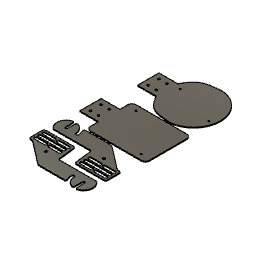
DécoupeCNC (Autodesk Fusion 360 design; units mm, degrees)
Autodesk Fusion 360 part; units mm, degrees
sketch "Esquisse2" plane through (0, 0, 0) normal (0, 0, 1) x (1, 0, 0) in component "Support Joystick v4"
  line L0 (0, 0) -> (-70, 0)
  circle A0 centre (100, 0) radius 82.5
  line L1 (250, 0) -> (-130, 0)
  spline S0 degree 5 poles (0, 20) (0, 22.4882) (0.1779, 27.4114) (0.975, 34.6277) (3.4457, 44.3914) (10.1068, 57.8847) (21.3924, 73.1358) (35.9935, 85.4932) (52.8737, 92.6951) (72.095, 96.3693) (93.5882, 98.471) (117.0022, 100.5708) (140.5192, 100.2508) (161.4884, 92.9068) (178.6566, 78.1832) (191.1793, 56.7401) (197.2314, 35.6259) (199.4965, 18.2943) (200, 6.1899) (200, 0) knots 0 0 0 0 0 0 0.066667 0.133333 0.2 0.266667 0.333333 0.4 0.466667 0.533333 0.6 0.666667 0.733333 0.8 0.866667 0.933333 1 1 1 1 1 1
  line L2 (0, 0) -> (0, 40)
  line L3 (96.4605, 99.786) -> (143.5395, 100.214)
  line L4 (4.3857, 52.2523) -> (35.6143, 87.7477)
  spline S1 degree 5 poles (0, -20) (0, -22.4882) (0.1779, -27.4114) (0.975, -34.6277) (3.4457, -44.3914) (10.1068, -57.8847) (21.3924, -73.1358) (35.9935, -85.4932) (52.8737, -92.6951) (72.095, -96.3693) (93.5882, -98.471) (117.0022, -100.5708) (140.5192, -100.2508) (161.4884, -92.9068) (178.6566, -78.1832) (191.1793, -56.7401) (197.2314, -35.6259) (199.4965, -18.2943) (200, -6.1899) (200, 0) knots 0 0 0 0 0 0 0.066667 0.133333 0.2 0.266667 0.333333 0.4 0.466667 0.533333 0.6 0.666667 0.733333 0.8 0.866667 0.933333 1 1 1 1 1 1
  line L5 (200, 30) -> (200, -30)
  line L6 (0, 0) -> (0, -40)
  line L7 (4.3857, -52.2523) -> (35.6143, -87.7477)
  line L8 (96.4605, -99.786) -> (143.5395, -100.214)
  line L9 (200, -30) -> (200, 30)
  circle A1 centre (22.2756, 27.6617) radius 3.1
  circle A2 centre (179.3345, -22.6338) radius 3.1
  ellipse E0 centre (100, 0) end of major axis (100, 100) minor radius 100
  line L10 (100, -100) -> (100, 100)
  line L11 (200, 0) -> (0, 0)
  line L12 (-70, 40) -> (0, 40)
  line L13 (0, 40) -> (0, -40)
  line L14 (0, -40) -> (-70, -40)
  line L15 (-70, -40) -> (-70, 40)
  line L16 (-70, 40) -> (0, -40) construction
  line L17 (0, 40) -> (-70, -40) construction
  line L18 (0, -40) -> (10.9445, -57.8049)
  line L19 (0, 40) -> (10.9445, 57.8049)
  line L20 (-20, -20) -> (-50, -20)
  line L21 (-50, -20) -> (-50, 20)
  line L22 (-50, 20) -> (-20, 20)
  line L23 (-20, 20) -> (-20, -20)
  circle A3 centre (-50, 20) radius 4
  circle A4 centre (-20, 20) radius 4
  circle A5 centre (-50, -20) radius 4
  circle A6 centre (-20, -20) radius 4
  point P0 (-35, 0)
  point P1 (20, 70)
  point P2 (120, 100)
  point P3 (20, -70)
  point P4 (120, -100)
  point P5 (-35, 0)
  dimension "d3_2" = 70
  dimension "d5_1" = 165
  dimension "d6_1" = 6.2
  dimension "d7_1" = 6.2
  dimension "d18_1" = 70
  dimension "d19_2" = 80
  dimension "d28" = 20
  dimension "d29" = 8
  dimension "d32" = 30
  dimension "d33" = -40
  constraint coincident L0.start L2.start
  constraint horizontal L0
  constraint midpoint L0 P5
  constraint coincident L1 S0.end
  constraint midpoint S0.start L2
  constraint perpendicular L0 L2
  constraint midpoint P2 L3
  constraint midpoint P1 L4
  constraint midpoint S0.end L5
  constraint symmetric S0.start L1 S1.start
  constraint symmetric L1 P1 P3
  constraint symmetric L1 P2 P4
  constraint symmetric L1 L0.start L2.start
  constraint symmetric L1 L2.end L6.end
  constraint symmetric L1 L3.start L8.start
  constraint symmetric L1 L3.end L8.end
  constraint symmetric L1 L4.start L7.start
  constraint symmetric L1 L4.end L7.end
  constraint symmetric L1 L5.start L5.end
  constraint symmetric L1 L5.end L5.start
  constraint coincident A0 A1.centre
  constraint coincident A0 A2.centre
  constraint coincident E0 L10.start
  constraint coincident E0 L10.end
  constraint coincident S0.end E0
  constraint coincident L0.start E0
  constraint concentric A0 E0
  constraint perpendicular L1 L10
  constraint horizontal L12
  constraint perpendicular L12 L13
  constraint parallel L12 L14
  constraint parallel L13 L15
  constraint coincident L16 P5
  constraint coincident L17 P5
  constraint coincident P5 P0
  constraint coincident S1 L18.end
  constraint coincident L2.end L12.end
  constraint coincident S0 L19.end
  constraint coincident L21.end L22.start
  measures "d3_2" distance of L0.start L0.end
  measures "d5_1" diameter of A0
  measures "d6_1" diameter of A2
  measures "d7_1" diameter of A1
  measures "d18_1" distance of L6.end L14.end
  measures "d19_2" distance of L2.end L6.end
  measures "d29" diameter of A3
extrude "Extrusion1" add sketch "Esquisse2" along normal blind 3 contours L0 L1 L6 L13 L14 L15 L20 L21 L23 A5 A6 | A0 L1 S0 A1 E0 L10 L11 | L0 L1 L2 L12 L13 L15 L21 L22 L23 A3 A4 | A0 L1 S0 E0 L10 L11 | A0 L1 S1 E0 L10 L11 | L0 L1 L20 L21 L23 A5 A6 | L0 L1 L21 L22 L23 A3 A4 | A0 L1 L10 L11 | A0 L1 A1 L10 L11 | A0 L1 A2 L10 L11 | A0 L1 S1 A2 E0 L10 L11 | A0 L1 L10 L11 makes body 1 in component "Support Joystick v4"
extrude "Extrusion2" cut sketch "Esquisse2" along normal blind 40 contours S1 E0 | S0 L3 E0 | S0 E0 | S1 L8 E0 bodies 1 in component "Support Joystick v4"
extrude "Extrusion3" add sketch "Esquisse2" along normal blind 3 contours S1 L6 E0 L13 L18 | S0 L2 E0 L13 L19 | S0 L2 L13 L19 | S1 L6 L13 L18 bodies 1 in component "Support Joystick v4"
sketch "Esquisse1" plane through (0, 0, 0) normal (0, 0, 1) x (1, 0, 0) in component "Support chaise Joystick v3"
  line L0 (56.5899, -2) -> (56.5899, -107.5251)
  line L1 (52.1537, -112.4932) -> (-9.5638, -119.4966)
  line L2 (-14, -124.4647) -> (-14, -263.5)
  line L3 (0.0899, -2) -> (0.0899, -2.5568)
  line L4 (-4.0699, -14.767) -> (-64.8402, -93.6035)
  line L5 (-69, -105.8137) -> (-69, -198.5386)
  arc A0 (52.1537, -112.4932) -> (56.5899, -107.5251) centre (51.5899, -107.5251) ccw
  arc A1 (-4.0699, -14.767) -> (0.0899, -2.5568) centre (-19.9101, -2.5568) ccw
  arc A2 (-64.8402, -93.6035) -> (-69, -105.8137) centre (-49, -105.8137) ccw
  circle A3 centre (-11.9332, -71.527) radius 4.5
  arc A4 (-41.6811, -245.7073) -> (-41.6811, -237.7073) centre (-41.6811, -241.7073) ccw
  arc A5 (-9.5638, -119.4966) -> (-14, -124.4647) centre (-9, -124.4647) ccw
  line L6 (7.0679, -8.5777) -> (7.0679, -46.452)
  arc A6 (7.0679, -46.452) -> (18.0679, -46.452) centre (12.5679, -46.452) ccw
  line L7 (18.0679, -46.452) -> (18.0679, -8.5777)
  arc A7 (18.0679, -8.5777) -> (7.0679, -8.5777) centre (12.5679, -8.5777) ccw
  line L8 (12.5679, -3.0777) -> (12.5679, -51.952) construction
  line L9 (38.0679, -8.5777) -> (38.0679, -46.452)
  arc A8 (38.0679, -46.452) -> (49.0679, -46.452) centre (43.5679, -46.452) ccw
  line L10 (49.0679, -46.452) -> (49.0679, -8.5777)
  arc A9 (49.0679, -8.5777) -> (38.0679, -8.5777) centre (43.5679, -8.5777) ccw
  line L11 (7.0679, -61.5777) -> (7.0679, -99.452)
  arc A10 (7.0679, -99.452) -> (18.0679, -99.452) centre (12.5679, -99.452) ccw
  line L12 (18.0679, -99.452) -> (18.0679, -61.5777)
  arc A11 (18.0679, -61.5777) -> (7.0679, -61.5777) centre (12.5679, -61.5777) ccw
  line L13 (49.0679, -99.452) -> (49.0679, -61.5777)
  arc A12 (49.0679, -61.5777) -> (38.0679, -61.5777) centre (43.5679, -61.5777) ccw
  arc A13 (38.0679, -99.452) -> (49.0679, -99.452) centre (43.5679, -99.452) ccw
  line L14 (38.0679, -61.5777) -> (38.0679, -99.452)
  line L15 (22.5679, -8.5777) -> (22.5679, -99.5777)
  arc A14 (22.5679, -99.5777) -> (33.5679, -99.5777) centre (28.0679, -99.5777) ccw
  line L16 (33.5679, -99.5777) -> (33.5679, -8.5777)
  arc A15 (33.5679, -8.5777) -> (22.5679, -8.5777) centre (28.0679, -8.5777) ccw
  line L17 (28.0679, -3.0777) -> (28.0679, -105.0777) construction
  line L18 (-41.6811, -237.7073) -> (-71.5558, -237.1789)
  line L19 (-41.6811, -245.7073) -> (-71.5558, -246.2356)
  arc A16 (-41.6811, -206.7073) -> (-75.3308, -232.0792) centre (-41.6811, -241.7073) ccw
  arc A17 (-75.3308, -251.3353) -> (-14, -263.1259) centre (-41.6811, -241.7073) ccw
  arc A18 (-75.3308, -232.0792) -> (-71.5558, -237.1789) centre (-71.4851, -233.1796) ccw
  arc A19 (-71.5558, -246.2356) -> (-75.3308, -251.3353) centre (-71.4851, -250.235) ccw
  arc A20 (-41.6811, -201.6751) -> (-74.8783, -219.3349) centre (-41.6811, -241.7073) ccw construction
  arc A21 (-41.6811, -206.7073) -> (-70.7053, -222.1472) centre (-41.6811, -241.7073) ccw
  arc A22 (-41.6811, -206.7073) -> (-41.6811, -196.643) centre (-41.6811, -201.6751) ccw
  arc A23 (-41.6811, -196.643) -> (-63.0989, -202.0579) centre (-41.6811, -241.7073) ccw
  arc A24 (-41.6811, -201.6751) -> (-74.8783, -219.3349) centre (-41.6811, -241.7073) ccw construction
  arc A25 (-69, -198.5386) -> (-63.0989, -202.0579) centre (-65, -198.5386) ccw
  line L20 (0.0899, -2) -> (0.0899, -1.3614)
  line L21 (5.0899, 3.6386) -> (51.5899, 3.6386)
  line L22 (56.5899, -1.3614) -> (56.5899, -3.9922)
  arc A26 (5.0899, 3.6386) -> (0.0899, -1.3614) centre (5.0899, -1.3614) ccw
  arc A27 (56.5899, -1.3614) -> (51.5899, 3.6386) centre (51.5899, -1.3614) ccw
  point P0 (0.0899, 3)
  point P1 (56.5899, 3)
  dimension "d3_1" = 56.5
  dimension "d5" = 20
  dimension "d6" = 9
  dimension "d7" = 70
  dimension "d10" = 5
  dimension "d11_1" = 11
  dimension "d12_1" = 11
  dimension "d13_1" = 11
  dimension "d14_1" = 11
  dimension "d15_1" = 11
  dimension "d16_1" = 4
  dimension "d17_1" = 4
  dimension "d19_1" = 4
  dimension "d22" = 5
  constraint parallel L3 L5
  constraint coincident P1 L0
  constraint coincident P0 L3
  constraint tangent L0 A0
  constraint tangent L1 A0
  constraint tangent L3 A1
  constraint tangent L4 A1
  constraint tangent L4 A2
  constraint tangent L5 A2
  constraint equal A1 A2
  constraint coincident L2 A17.end
  constraint tangent L1 A5
  constraint tangent L2 A5
  constraint tangent L6 A6
  constraint tangent A6 L7
  constraint parallel L6 L7
  constraint tangent L7 A7
  constraint tangent L6 A7
  constraint midpoint A7 L8.start
  constraint midpoint A6 L8.end
  constraint vertical L8
  constraint tangent L9 A8
  constraint tangent A8 L10
  constraint parallel L9 L10
  constraint tangent L10 A9
  constraint tangent L9 A9
  constraint tangent L11 A10
  constraint tangent A10 L12
  constraint parallel L11 L12
  constraint tangent L12 A11
  constraint tangent L11 A11
  constraint tangent A13 L14
  constraint tangent L13 A13
  constraint parallel L13 L14
  constraint tangent L13 A12
  constraint tangent A12 L14
  constraint tangent L15 A14
  constraint tangent A14 L16
  constraint parallel L15 L16
  constraint tangent L16 A15
  constraint tangent L15 A15
  constraint midpoint A15 L17.start
  constraint midpoint A14 L17.end
  constraint concentric A16 A17
  constraint tangent L18 A18
  constraint tangent A16 A18
  constraint tangent L19 A19
  constraint tangent A17 A19
  constraint coincident A4.centre A16.centre
  constraint tangent A21 A22
  constraint tangent A22 A23
  constraint coincident A20.end A24.end
  constraint coincident A20.start A22.centre
  constraint tangent A23 A25
  constraint tangent L5 A25
  constraint perpendicular L0 L21
  constraint coincident L0 L22.end
  constraint perpendicular L21 L22
  constraint tangent L20 A26
  constraint tangent L21 A26
  constraint tangent L21 A27
  constraint tangent L22 A27
  constraint equal A26 A27
  measures "d3_1" distance of P0 P1
  measures "d5" radius of A1
  measures "d6" diameter of A3
  measures "d7" diameter of A16
  measures "d10" radius of A5
  measures "d11_1" diameter of A6
  measures "d12_1" diameter of A8
  measures "d13_1" diameter of A10
  measures "d14_1" diameter of A13
  measures "d15_1" diameter of A14
  measures "d16_1" radius of A18
  measures "d17_1" radius of A19
  measures "d19_1" radius of A25
  measures "d22" radius of A26
extrude "Extrusion1'" add sketch "Esquisse1" along normal blind 3 separate body makes body 2 in component "Support chaise Joystick v3"
ref_plane "Plan de construction1" through (100, 0, 0) normal (1, 0, 0) x (0, 1, 0) in component "Support chaise Joystick v3"
mirror "Symétrie miroir1" about plane through (100, 0, 0) normal (1, 0, 0) of bodies 2 makes body 3 in component "Support chaise Joystick v3"
sketch "Esquisse1 (2)" plane through (0, 0, 0) normal (0, 0, 1) x (1, 0, 0) in component "Support Throttle v3"
  circle A0 centre (-65, 59.5) radius 3.2016
  circle A1 centre (85, -71) radius 3.1623
  line L0 (-85, 79.25) -> (105, 79.25)
  line L1 (120, 64.25) -> (120, -75.75)
  line L2 (105, -90.75) -> (-85, -90.75)
  line L3 (-100, -75.75) -> (-100, 64.25)
  line L4 (-100, -5.75) -> (-170, -5.75)
  line L5 (-170, 34.25) -> (-100, 34.25)
  line L6 (-100, 34.25) -> (-100, -45.75)
  line L7 (-100, -45.75) -> (-170, -45.75)
  line L8 (-170, -45.75) -> (-170, 34.25)
  line L9 (-170, 34.25) -> (-100, -45.75) construction
  line L10 (-100, 34.25) -> (-170, -45.75) construction
  arc A2 (-85, 79.25) -> (-100, 64.25) centre (-85, 64.25) ccw
  arc A3 (120, 64.25) -> (105, 79.25) centre (105, 64.25) ccw
  arc A4 (105, -90.75) -> (120, -75.75) centre (105, -75.75) ccw
  arc A5 (-100, -75.75) -> (-85, -90.75) centre (-85, -75.75) ccw
  line L11 (-150, -25.75) -> (-150, 14.25)
  line L12 (-150, 14.25) -> (-120, 14.25)
  line L13 (-120, 14.25) -> (-120, -25.75)
  line L14 (-120, -25.75) -> (-150, -25.75)
  circle A6 centre (-150, 14.25) radius 4
  circle A7 centre (-120, 14.25) radius 4
  circle A8 centre (-150, -25.75) radius 4
  circle A9 centre (-120, -25.75) radius 4
  point P0 (120, 79.25)
  point P1 (120, -90.75)
  point P2 (10, -5.75)
  point P3 (-135, -5.75)
  dimension "d1" = 170
  dimension "d2" = 70
  dimension "d3" = 70
  dimension "d4" = 80
  dimension "d11" = 15
  dimension "d14" = 20
  dimension "d15" = 8
  dimension "d18" = 30
  dimension "d19" = -40
  constraint horizontal L0
  constraint perpendicular L0 L1
  constraint parallel L0 L2
  constraint parallel L1 L3
  constraint perpendicular L3 L4
  constraint horizontal L5
  constraint perpendicular L5 L6
  constraint parallel L5 L7
  constraint parallel L6 L8
  constraint coincident L9 P3
  constraint coincident L10 P3
  constraint midpoint L4 P3
  constraint coincident L3 L4.start
  constraint tangent L0 A2
  constraint tangent L3 A2
  constraint coincident P0 L0
  constraint coincident P0 L1
  constraint tangent L0 A3
  constraint tangent L1 A3
  constraint equal A2 A3
  constraint coincident P1 L1
  constraint coincident P1 L2
  constraint tangent L1 A4
  constraint tangent L2 A4
  constraint equal A2 A4
  constraint tangent L2 A5
  constraint tangent L3 A5
  constraint equal A2 A5
  constraint coincident L11.end L12.start
  measures "d1" distance of P0 P1
  measures "d2" distance of L4.start L4.end
  measures "d3" distance of L6.end L7.end
  measures "d4" distance of L5.end L6.end
  measures "d11" radius of A2
  measures "d15" diameter of A6
extrude "Extrusion1''" add sketch "Esquisse1 (2)" along normal blind 3 separate body makes body 4 in component "Support Throttle v3"
extrude "Extrusion2'" cut sketch "Esquisse1 (2)" along normal blind 3 contours L12 L13 A7 | L12 L13 A7 | L13 L14 A9 | L13 L14 A9 | L11 L14 A8 | L11 L14 A8 | L11 L12 A6 | L11 L12 A6 bodies 4 in component "Support Throttle v3"
sketch "Esquisse1 (3)" plane through (0, 0, 3) normal (0, 0, 1) x (-1, 0, 0)
  circle A0 centre (-22.2756, -187.6617) radius 3.1
  circle A1 centre (-179.3345, -137.3662) radius 3.1
  circle A2 centre (50, -180) radius 4
  circle A3 centre (20, -180) radius 4
  circle A4 centre (50, -140) radius 4
  circle A5 centre (20, -140) radius 4
  line L0 (70, -200) -> (70, -120)
  line L1 (70, -120) -> (0, -120)
  line L2 (0, -120) -> (-10.9445, -102.1951)
  spline S0 degree 5 poles (-10.9445, -102.1951) (-11.0037, -102.0999) (-12.8345, -99.1697) (-16.8813, -93.3048) (-24.2145, -84.4758) (-35.7697, -74.6962) (-48.9808, -68.9675) (-59.8244, -66.2242) (-67.3838, -64.8492) (-71.1083, -64.2646) knots 0.19776 0.19776 0.19776 0.19776 0.19776 0.19776 0.2 0.266667 0.333333 0.4 0.461557 0.461557 0.461557 0.461557 0.461557 0.461557
  spline S1 degree 5 poles (-71.1083, -64.2646) (-71.4175, -64.2161) (-75.7696, -63.5418) (-82.9723, -62.6189) (-90.499, -61.8591) (-98.3193, -61.1267) (-105.9435, -60.582) (-108.9719, -60.4033) knots 0.461557 0.461557 0.461557 0.461557 0.461557 0.461557 0.466667 0.533333 0.576912 0.576912 0.576912 0.576912 0.576912 0.576912
  arc A6 (-108.9719, -60.4033) -> (-108.9719, -259.5967) centre (-100, -160) ccw
  spline S2 degree 5 poles (-108.9719, -259.5967) (-105.9435, -259.418) (-98.3193, -258.8733) (-90.499, -258.1409) (-82.9723, -257.3811) (-75.7696, -256.4582) (-71.4175, -255.7839) (-71.1083, -255.7354) knots -0.576912 -0.576912 -0.576912 -0.576912 -0.576912 -0.576912 -0.533333 -0.466667 -0.461557 -0.461557 -0.461557 -0.461557 -0.461557 -0.461557
  spline S3 degree 5 poles (-71.1083, -255.7354) (-67.3838, -255.1508) (-59.8244, -253.7758) (-48.9808, -251.0325) (-35.7697, -245.3038) (-24.2145, -235.5242) (-16.8813, -226.6952) (-12.8345, -220.8303) (-11.0037, -217.9001) (-10.9445, -217.8049) knots -0.461557 -0.461557 -0.461557 -0.461557 -0.461557 -0.461557 -0.4 -0.333333 -0.266667 -0.2 -0.19776 -0.19776 -0.19776 -0.19776 -0.19776 -0.19776
  line L3 (-10.9445, -217.8049) -> (0, -200)
  line L4 (0, -200) -> (70, -200)
  line L5 (-250, -250) -> (-750, -250)
  line L6 (-750, -250) -> (-750, 250)
  line L7 (-750, 250) -> (-250, 250)
  line L8 (-250, 250) -> (-250, -250)
  constraint horizontal L5
  constraint vertical L6
  constraint horizontal L7
  constraint vertical L8
move_body "Déplacer1" bodies 3 to x (1, 0, 0) y (0, 1, 0) z (0, 0, 1) at (425, 225, 0) in component "Support chaise Joystick v3"
move_body "Déplacer2" bodies 2 to x (0, -1, 0) y (1, 0, 0) z (0, 0, 1) at (526.2222, -227.1924, 0) in component "Support chaise Joystick v3"
move_body "Déplacer3" bodies 3 to x (1, 0, 0) y (0, 1, 0) z (0, 0, 1) at (-10, 0, 0) in component "Support chaise Joystick v3"
move_body "Déplacer4" bodies 2 to x (1, 0, 0) y (0, 1, 0) z (0, 0, 1) at (0, 10, 0) in component "Support chaise Joystick v3"
move_body "Déplacer5" bodies 3 to x (0, -1, 0) y (-1, 0, 0) z (0, 0, -1) at (476.7028, 336.7028, 0) in component "Support chaise Joystick v3"
move_body "Aligner1" bodies 3 to x (1, 0, 0) y (0, 1, 0) z (0, 0, 1) at (0, 0, 3) in component "Support chaise Joystick v3"
component "Support chaise Joystick v3" placed x (1, 0, 0) y (0, 1, 0) z (0, 0, 1) at (0, 0, 0)
component "Support Throttle v3" placed x (1, 0, 0) y (0, 1, 0) z (0, 0, 1) at (-200, 0, 0)
component "Support Joystick v4" placed x (1, 0, 0) y (0, 1, 0) z (0, 0, 1) at (0, 160, 0)
